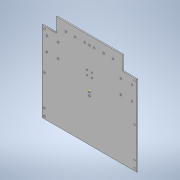
# Autodesk Inventor part: 20220522
Saved by Autodesk Inventor 2020 (Build 240168000, 168)
## iProperties
Created: 2022-05-21
Part Number: 20220522
Material: 一般
Document SubType Name: Modeling
Designer: Naggy
Density: 1 g/cm^3
Appearance: 既定
Author: Naggy
Autodesk Inventor part; units mm, degrees
ref_plane "YZ Plane" through (0, 0, 0) normal (1, 0, 0) x (0, 1, 0)
ref_plane "XZ Plane" through (0, 0, 0) normal (0, 1, 0) x (-1, 0, 0)
ref_plane "XY Plane" through (0, 0, 0) normal (0, 0, 1) x (1, 0, 0)
sketch "スケッチ1" plane through (0, 0, 0) normal (0, 0, 1) x (1, 0, 0)
  line L0 (-100, -100) -> (100, -100)
  line L1 (100, -100) -> (100, 100)
  line L2 (100, 100) -> (-100, 100)
  line L3 (-100, 100) -> (-100, -100)
  line L4 (-100, -100) -> (100, 100) construction
  line L5 (100, -100) -> (-100, 100) construction
  point P0 (0, 0)
  dimension "d0" = 200
  dimension "d1" = 200
  constraints: 12 end point, 2 midpoint, 2 parallel, 1 horizontal, 1 perpendicular
  measures "d0" distance between parallel lines of L1 L3
  measures "d1" distance between parallel lines of L0 L2
extrude "押し出し1" add sketch "スケッチ1" along normal blind 2
sketch "スケッチ2" plane through (0, 0, 2) normal (0, 0, 1) x (1, 0, 0)
  line L0 (100, 100) -> (-100, 100) projected
  line L1 (100, 100) -> (70, 100)
  line L2 (70, 100) -> (70, 70)
  line L3 (70, 70) -> (100, 70)
  line L4 (100, 70) -> (100, 100)
  line L5 (-100, -100) -> (100, -100) projected
  line L6 (-100, 100) -> (-100, -100) projected
  line L7 (-100, 100) -> (-70, 100)
  line L8 (-70, 100) -> (-70, 70)
  line L9 (-70, 70) -> (-100, 70)
  line L10 (-100, 70) -> (-100, 100)
  point P0 (0, 0)
  point P1 (-100, 70)
  dimension "d4" = 170
  dimension "d5" = 30
  dimension "d6" = 30
  dimension "d7" = 170
  constraints: 16 end point, 4 parallel, 2 horizontal, 2 perpendicular
  measures "d4" distance between parallel lines of L3 L5
  measures "d5" distance between parallel lines of L4 L2
  measures "d6" distance between parallel lines of L8 L6
  measures "d7" distance between parallel lines of L9 L5
extrude "押し出し2" cut sketch "スケッチ2" against normal blind 2
sketch "スケッチ3" plane through (0, 0, 0) normal (0, 0, -1) x (-1, 0, 0)
  line L0 (-70, 100) -> (70, 100) projected
  point P0 (0, 0)
  point P1 (-35.7932, 78)
  point P2 (37.7411, 78)
  point P3 (-61, 89.1596)
  point P4 (61, 89.1596)
  point P5 (-50, 82.5)
  point P6 (-30, 82.5)
  point P7 (-10, 82.5)
  point P8 (0.0001, 82.5183)
  point P9 (10, 82.5545)
  point P10 (30, 82.5545)
  point P11 (50, 82.5545)
  point P12 (51.6496, 93.6869)
  dimension "d10" = 22
  dimension "d11" = 61
  dimension "d12" = 61
  dimension "d13" = 17.5
  dimension "d14" = 11
  dimension "d15" = 31
  dimension "d16" = 51
  dimension "d17" = 71
  dimension "d18" = 91
  dimension "d19" = 111
  measures "d10" distance from line of point (-35.793, 78) L0
  measures "d11" horizontal distance of point (0, 0) point (-61, 89.16)
  measures "d12" horizontal distance of point (61, 89.16) point (0, 0)
  measures "d13" distance from line of point (-50, 82.5) L0
  measures "d14" horizontal distance of point (-50, 82.5) point (-61, 89.16)
  measures "d15" horizontal distance of point (-30, 82.5) point (-61, 89.16)
  measures "d16" horizontal distance of point (-10, 82.5) point (-61, 89.16)
  measures "d17" horizontal distance of point (10, 82.555) point (-61, 89.16)
  measures "d18" horizontal distance of point (30, 82.555) point (-61, 89.16)
  measures "d19" horizontal distance of point (50, 82.555) point (-61, 89.16)
hole "穴1" at (50, 82.5, 0) at (30, 82.5, 0) at (10, 82.5, 0) at (-10, 82.5545, 0) at (-30, 82.5545, 0) at (-50, 82.5545, 0) at (-0.0001, 82.5183, 0) direction (0, 0, 1) diameter 3.4 end through all clearance for "Flat Head Machine Screw" size "M3" standard "Ansi Metric M Profile"
sketch "スケッチ4" plane through (0, 0, 0) normal (0, 0, -1) x (-1, 0, 0)
  line L0 (-70, 70) -> (-100, 70) projected
  line L1 (-100, -100) -> (-100, 70) projected
  line L2 (100, 70) -> (100, -100) projected
  line L3 (100, 70) -> (70, 70) projected
  point P0 (0, 0)
  point P1 (-90, 55)
  point P2 (-66, 55)
  point P3 (-90, 25)
  point P4 (-66, 25)
  point P5 (90, 58)
  point P6 (66, 58)
  point P7 (90, 12.16)
  point P8 (66, 12.16)
  dimension "d27" = 15
  dimension "d28" = 15
  dimension "d29" = 10
  dimension "d30" = 24
  dimension "d31" = 10
  dimension "d32" = 30
  dimension "d33" = 30
  dimension "d34" = 24
  dimension "d35" = 10
  dimension "d36" = 12
  dimension "d37" = 24
  dimension "d38" = 10
  dimension "d39" = 24
  measures "d27" distance from line of point (-90, 55) L0
  measures "d28" distance from line of point (-66, 55) L0
  measures "d29" distance from line of point (-90, 55) L1
  measures "d30" distance of point (-66, 55) point (-90, 55)
  measures "d31" distance from line of point (-90, 25) L1
  measures "d32" distance of point (-90, 25) point (-90, 55)
  measures "d33" distance of point (-66, 25) point (-66, 55)
  measures "d34" distance of point (-66, 25) point (-90, 25)
  measures "d35" distance from line of point (90, 58) L2
  measures "d36" distance from line of point (90, 58) L3
  measures "d37" distance of point (66, 58) point (90, 58)
  measures "d38" distance from line of point (90, 12.16) L2
  measures "d39" distance of point (66, 12.16) point (90, 12.16)
hole "穴2" at (66, 25, 0) at (90, 25, 0) at (66, 55, 0) at (90, 55, 0) direction (0, 0, 1) diameter 3.4 end through all clearance for "Flat Head Machine Screw" size "M3" standard "Ansi Metric M Profile"
sketch "スケッチ5" plane through (0, 0, 0) normal (0, 0, -1) x (-1, 0, 0)
  point P0 (0, 0)
sketch "スケッチ6" plane through (0, 0, 0) normal (0, 0, -1) x (-1, 0, 0)
  line L0 (100, 70) -> (70, 70) projected
  line L1 (100, 70) -> (100, -100) projected
  point P0 (0, 0)
  point P1 (90, 55)
  point P2 (66, 55)
  point P3 (90, 25)
  point P4 (66, 25)
  dimension "d47" = 15
  dimension "d48" = 15
  dimension "d49" = 10
  dimension "d50" = 24
  dimension "d51" = 10
  dimension "d52" = 24
  dimension "d53" = 30
  dimension "d54" = 30
  measures "d47" distance from line of point (90, 55) L0
  measures "d48" distance from line of point (66, 55) L0
  measures "d49" distance from line of L1 point (90, 55)
  measures "d50" distance of point (66, 55) point (90, 55)
  measures "d51" distance from line of point (90, 25) L1
  measures "d52" distance of point (66, 25) point (90, 25)
  measures "d53" distance of point (90, 25) point (90, 55)
  measures "d54" distance of point (66, 25) point (66, 55)
hole "穴3" at (-90, 25, 0) at (-66, 25, 0) at (-66, 55, 0) at (-90, 55, 0) direction (0, 0, 1) diameter 3.4 end through all clearance for "Flat Head Machine Screw" size "M3" standard "Ansi Metric M Profile"
sketch "スケッチ7" plane through (0, 0, 0) normal (0, 0, -1) x (-1, 0, 0)
  point P0 (0, 0)
sketch "スケッチ8" plane through (0, 0, 0) normal (0, 0, -1) x (-1, 0, 0)
  line L0 (-100, -100) -> (-100, 70) projected
  line L1 (-70, 70) -> (-100, 70) projected
  line L2 (100, 70) -> (70, 70) projected
  line L3 (100, 70) -> (100, -100) projected
  point P0 (0, 0)
  point P1 (-95, 65)
  point P2 (95, 65)
  dimension "d62" = 5
  dimension "d63" = 5
  dimension "d64" = 5
  dimension "d65" = 5
  measures "d62" distance from line of point (-95, 65) L0
  measures "d63" distance from line of point (-95, 65) L1
  measures "d64" distance from line of point (95, 65) L2
  measures "d65" distance from line of point (95, 65) L3
hole "穴4" at (95, 65, 0) at (-95, 65, 0) direction (0, 0, 1) diameter 3.4 end through all clearance for "Flat Head Machine Screw" size "M3" standard "Ansi Metric M Profile"
sketch "スケッチ9" plane through (0, 0, 0) normal (0, 0, -1) x (-1, 0, 0)
  line L0 (-100, -100) -> (-100, 70) projected
  line L1 (100, -100) -> (-100, -100) projected
  line L2 (100, 70) -> (100, -100) projected
  point P0 (0, 0)
  point P1 (-95, -95)
  point P2 (95, -95)
  dimension "d73" = 5
  dimension "d74" = 5
  dimension "d75" = 5
  dimension "d76" = 5
  measures "d73" distance from line of point (-95, -95) L0
  measures "d74" distance from line of L1 point (-95, -95)
  measures "d75" distance from line of point (95, -95) L1
  measures "d76" distance from line of point (95, -95) L2
hole "穴5" at (95, -95, 0) at (-95, -95, 0) direction (0, 0, 1) diameter 3.4 end through all clearance for "Flat Head Machine Screw" size "M3" standard "Ansi Metric M Profile"
sketch "スケッチ10" plane through (0, 0, 0) normal (0, 0, -1) x (-1, 0, 0)
  circle A0 centre (-95, 65) radius 1.7 projected
  line L0 (-100, -100) -> (-100, 70) projected
  line L1 (100, 70) -> (100, -100) projected
  point P0 (0, 0)
  point P1 (-95, -15)
  point P2 (95, -25)
  dimension "d84" = 80
  dimension "d85" = 5
  dimension "d86" = 5
  measures "d84" distance of point (-95, -15) A0.centre
  measures "d85" distance from line of point (-95, -15) L0
  measures "d86" distance from line of point (95, -25) L1
hole "穴6" at (95, -15, 0) direction (0, 0, 1) diameter 3.4 end through all clearance for "Flat Head Machine Screw" size "M3" standard "Ansi Metric M Profile"
sketch "スケッチ11" plane through (0, 0, 0) normal (0, 0, -1) x (-1, 0, 0)
  line L0 (-70, 100) -> (70, 100) projected
  point P0 (0, 0)
  point P1 (0, 0)
  point P2 (0, -10)
  dimension "d94" = 110
  constraints: 1 coincident
  measures "d94" distance from line of point (0, -10) L0
hole "穴7" at (0, -10, 0) direction (0, 0, 1) diameter 3.4 end through all clearance for "Flat Head Machine Screw" size "M3" standard "Ansi Metric M Profile"
sketch "スケッチ12" plane through (0, 0, 0) normal (0, 0, -1) x (-1, 0, 0)
  line L0 (100, -100) -> (-100, -100) projected
  line L1 (100, 70) -> (100, -100) projected
  line L2 (-100, -100) -> (-100, 70) projected
  point P0 (0, 0)
  point P1 (-95, -80)
  point P2 (95, -80)
  dimension "d102" = 20
  dimension "d103" = 20
  dimension "d104" = 5
  dimension "d105" = 5
  measures "d102" distance from line of point (-95, -80) L0
  measures "d103" distance from line of L0 point (95, -80)
  measures "d104" distance from line of point (95, -80) L1
  measures "d105" distance from line of point (-95, -80) L2
hole "穴8" at (95, -80, 0) at (-95, -80, 0) direction (0, 0, 1) diameter 3.4 end through all clearance for "Flat Head Machine Screw" size "M3" standard "Ansi Metric M Profile"
sketch "スケッチ13" plane through (0, 0, 0) normal (0, 0, -1) x (-1, 0, 0)
  point P0 (0, 0)
sketch "スケッチ14" plane through (0, 0, 0) normal (0, 0, -1) x (-1, 0, 0)
  line L0 (100, 70) -> (100, -100) projected
  circle A0 centre (95, 65) radius 1.7 projected
  point P0 (0, 0)
  point P1 (95, -15)
  dimension "d113" = 5
  dimension "d114" = 80
  measures "d113" distance from line of point (95, -15) L0
  measures "d114" distance of point (95, -15) A0.centre
hole "穴9" at (-95, -15, 0) direction (0, 0, 1) diameter 3.4 end through all clearance for "Flat Head Machine Screw" size "M3" standard "Ansi Metric M Profile"
sketch "スケッチ15" plane through (0, 0, 0) normal (0, 0, -1) x (-1, 0, 0)
  circle A0 centre (0, -10) radius 1.7 projected
  point P0 (0, 0)
  point P1 (0, -3)
  dimension "d122" = 7
  measures "d122" distance of point (0, -3) A0.centre
hole "穴10" at (0, -3, 0) direction (0, 0, 1) diameter 3.4 end through all clearance for "Flat Head Machine Screw" size "M3" standard "Ansi Metric M Profile"
sketch "スケッチ16" plane through (0, 0, 2) normal (0, 0, 1) x (1, 0, 0)
  point P0 (0, 0)
  point P1 (-5, 24.9689)
  point P2 (5, 25)
  point P3 (5, 35)
  point P4 (-5, 34.9689)
  dimension "d130" = 5
  dimension "d131" = 5
  dimension "d132" = 10
  dimension "d133" = 10
  dimension "d134" = 5
  dimension "d135" = 5
  measures "d130" horizontal distance of point (0, 0) point (-5, 24.969)
  measures "d131" horizontal distance of point (0, 0) point (5, 25)
  measures "d132" distance of point (5, 35) point (5, 25)
  measures "d133" distance of point (-5, 34.969) point (-5, 24.969)
  measures "d134" horizontal distance of point (0, 0) point (-5, 34.969)
  measures "d135" horizontal distance of point (0, 0) point (5, 35)
hole "穴11" at (-5, 34.9689, 2) at (-5, 24.9689, 2) at (5, 25, 2) at (5, 35, 2) direction (0, 0, -1) diameter 2.459 depth 8.8 tip angle 118 thread size "M3x0.5" class "6H" standard "ANSI Metric M Profile"
sketch "スケッチ17" plane through (0, 0, 2) normal (0, 0, 1) x (1, 0, 0)
  point P0 (0, 0)
